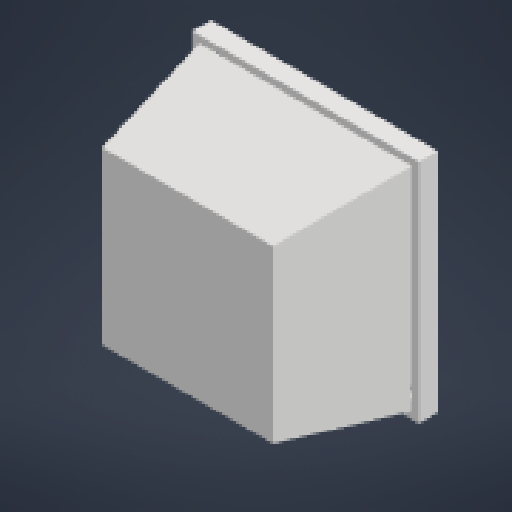
# Autodesk Inventor part: KeySwitch
Saved by Autodesk Inventor 2024.2 (Build 282272000, 272)
## iProperties
Created: 2023-11-23
Part Number: KeySwitch
Material: 일반
Document SubType Name: Modeling
Designer: 6gioc
Density: 1 g/cm^3
Appearance: 기본값
Author: 6gioc
Autodesk Inventor part; units mm, degrees
ref_plane "YZ Plane" through (0, 0, 0) normal (1, 0, 0) x (0, 1, 0)
ref_plane "XZ Plane" through (0, 0, 0) normal (0, 1, 0) x (-1, 0, 0)
ref_plane "XY Plane" through (0, 0, 0) normal (0, 0, 1) x (1, 0, 0)
sketch "스케치1" plane through (0, 0, 0) normal (0, 0, 1) x (1, 0, 0)
  circle A0 centre (-80.3814, -83.6055) radius 3 projected
  circle A1 centre (-80.3814, -83.6055) radius 1.5 projected
  circle A2 centre (-95.5814, -68.4055) radius 3 projected
  circle A3 centre (-95.5814, -68.4055) radius 1.5 projected
  line L0 (-78.3814, -66.4055) -> (-97.5814, -66.4055)
  line L1 (-97.5814, -66.4055) -> (-97.5814, -85.6055)
  line L2 (-97.5814, -85.6055) -> (-78.3814, -85.6055)
  line L3 (-78.3814, -85.6055) -> (-78.3814, -66.4055)
  point P0 (0, 0)
  dimension "d0" = 19.2
  dimension "d1" = 19.2
  dimension "d2" = 2
  dimension "d3" = 2
  constraints: 8 end point, 2 parallel, 1 horizontal, 1 perpendicular
  measures "d0" distance of L2.end L1.end
  measures "d1" distance of L1.end L0.end
  measures "d2" distance from line of L0 A3.centre
  measures "d3" distance from line of A1.centre L3
extrude "돌출1" add sketch "스케치1" along normal blind 1.6 contours L3 L2 A0 | A0 L2 L1 A2 L0 L3 | A2 L1 L0 picked at (-80.5204, -85.4352) picked at (-95.563, -66.5758)
sketch "스케치2" plane through (0, 0, 1.6) normal (0, 0, 1) x (1, 0, 0)
  line L0 (-78.9814, -67.0055) -> (-96.9814, -67.0055)
  line L1 (-96.9814, -67.0055) -> (-96.9814, -85.0055)
  line L2 (-96.9814, -85.0055) -> (-78.9814, -85.0055)
  line L3 (-78.9814, -85.0055) -> (-78.9814, -67.0055)
  line L4 (-97.5814, -85.6055) -> (-78.3814, -85.6055) projected
  line L5 (-78.3814, -85.6055) -> (-78.3814, -66.4055) projected
  line L6 (-78.3814, -66.4055) -> (-97.5814, -66.4055) projected
  line L7 (-97.5814, -66.4055) -> (-97.5814, -85.6055) projected
  circle A0 centre (-80.3814, -83.6055) radius 1.5 projected
  circle A1 centre (-95.5814, -68.4055) radius 1.5 projected
  point P0 (0, 0)
  dimension "d6" = 18
  dimension "d7" = 18
  dimension "d8" = 19.2
  dimension "d9" = 0.6
  dimension "d10" = 0.6
  constraints: 8 end point, 2 parallel, 1 horizontal, 1 perpendicular
  measures "d6" distance of L2.end L1.end
  measures "d7" distance of L1.end L0.end
  measures "d8" distance between parallel lines of L4 L6
  measures "d9" distance between parallel lines of L6 L0
  measures "d10" distance between parallel lines of L5 L3
extrude "돌출2" add sketch "스케치2" along normal blind 5 contours L3 A0 L2 L1 A1 L0 | A1 L1 L0 | L3 A0 L2 | A1 L1 L0 | L3 L2 A0
sketch "스케치3" plane through (0, 0, 6.6) normal (0, 0, 1) x (1, 0, 0)
  line L0 (-96.9814, -85.0055) -> (-78.9814, -85.0055) projected
  line L1 (-78.9814, -85.0055) -> (-78.9814, -67.0055) projected
  line L2 (-78.9814, -67.0055) -> (-96.9814, -67.0055) projected
  line L3 (-96.9814, -67.0055) -> (-96.9814, -85.0055) projected
  point P0 (0, 0)
extrude "돌출3" add sketch "스케치3" along normal blind 10 draft -10
